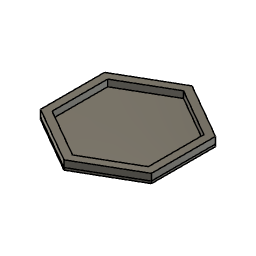
hexagon plate1 v8 (Autodesk Fusion 360 design; units mm, degrees)
Autodesk Fusion 360 part; units mm, degrees
note: some values were not read from the file. Set by a fixed rule: which sketch regions a step uses.
sketch "bottom of the plate" plane through (0, 0, 0) normal (0, 1, 0) x (1, 0, 0)
  line L0 (-150, -86.6025) -> (0, -173.2051)
  line L1 (0, -173.2051) -> (150, -86.6025)
  line L2 (150, -86.6025) -> (150, 86.6025)
  line L3 (150, 86.6025) -> (0, 173.2051)
  line L4 (0, 173.2051) -> (-150, 86.6025)
  line L5 (-150, 86.6025) -> (-150, -86.6025)
  line L6 (-150, 86.6025) -> (0, 0)
  line L7 (0, 0) -> (150, 86.6025)
  line L8 (0, 0) -> (0, -173.2051)
  dimension "d1" = 300
  dimension "d2" = 346.4102
  constraint coincident L6.end L7.start
  measures "d1" distance of L2 L5
  measures "d2" distance of L0.end L3.end
extrude "Extrude1" add sketch "bottom of the plate" along normal blind 6 makes body 1
sketch "sidePart" plane through (0, 6, 0) normal (0, 1, 0) x (-1, 0, 0)
  line L0 (150, -86.6025) -> (150, 86.6025)
  line L1 (150, 86.6025) -> (0, 173.2051)
  line L2 (0, 173.2051) -> (-150, 86.6025)
  line L3 (-150, 86.6025) -> (-150, -86.6025)
  line L4 (-150, -86.6025) -> (0, -173.2051)
  line L5 (0, -173.2051) -> (150, -86.6025)
  line L6 (-325.0555, -130) -> (-174.9445, -130)
  line L7 (-336.6025, -150) -> (-163.3975, -150)
  line L8 (-336.6025, -150) -> (-325.0555, -130)
  line L9 (-163.3975, -150) -> (-174.9445, -130)
extrude "Extrude2" add sketch "sidePart" along normal blind 6 separate body contours L0 L1 L2 L3 L4 L5 makes body 2
sketch "side" plane through (0, 6, 0) normal (0, 1, 0) x (-1, 0, 0)
  line L0 (-130, -75.0555) -> (0, -150.1111)
  line L1 (0, -150.1111) -> (130, -75.0555)
  line L2 (130, -75.0555) -> (130, 75.0555)
  line L3 (130, 75.0555) -> (0, 150.1111)
  line L4 (0, 150.1111) -> (-130, 75.0555)
  line L5 (-130, 75.0555) -> (-130, -75.0555)
  line L6 (-150, -86.6025) -> (0, -173.2051)
  line L7 (0, -173.2051) -> (150, -86.6025)
  line L8 (150, -86.6025) -> (150, 86.6025)
  line L9 (150, 86.6025) -> (0, 173.2051)
  line L10 (0, 173.2051) -> (-150, 86.6025)
  line L11 (-150, 86.6025) -> (-150, -86.6025)
  dimension "d9" = 130
  measures "d9" distance of origin L5
extrude "Extrude3" add sketch "side" along normal blind 12 bodies 1
sketch "Sketch5" plane through (-65, 0, 112.5833) normal (0.5, 0, -0.866025) x (-0.866025, 0, -0.5)
  line L0 (-75.0555, 6) -> (75.0555, 6)
  line L1 (75.0555, 6) -> (75.0555, 18)
  line L2 (75.0555, 18) -> (-75.0555, 18)
  line L3 (-75.0555, 18) -> (-75.0555, 6)
  dimension "d12" = 8
sketch "Sketch6" plane through (75, 0, -129.9038) normal (0.5, 0, -0.866025) x (-0.866025, 0, -0.5)
  line L0 (-86.6025, 0) -> (86.6025, 0)
  line L1 (86.6025, 0) -> (86.6025, 18)
  line L2 (86.6025, 18) -> (-86.6025, 18)
  line L3 (-86.6025, 18) -> (-86.6025, 0)
  dimension "d13" = 12
move_face "OffsetFaces1" offset 70 1 faces at (50, 18, -136.6396) on bodies 1
sketch "Sketch7" plane through (-130, 0, 0) normal (1, 0, 0) x (0, 0, -1)
  line L0 (-75.0555, 6) -> (75.0555, 6)
  line L1 (75.0555, 6) -> (75.0555, 88)
  line L2 (75.0555, 88) -> (-75.0555, 88)
  line L3 (-75.0555, 88) -> (-75.0555, 6)
  line L4 (-173.2051, 88) -> (-86.6025, 88)
  line L5 (-173.2051, 0) -> (-86.6025, 0)
  line L6 (-173.2051, 0) -> (-173.2051, 88)
  line L7 (173.2051, 0) -> (173.2051, 88)
  dimension "d15" = 17
  dimension "d16" = 346.4102
  measures "d16" distance of L6 L7
sketch "all_sides" plane through (0, 12, 0) normal (0, 1, 0) x (-1, 0, 0)
  line L0 (0, -173.2051) -> (150, -86.6025)
  line L1 (150, -86.6025) -> (150, 86.6025)
  line L2 (150, 86.6025) -> (0, 173.2051)
  line L3 (0, 173.2051) -> (-150, 86.6025)
  line L4 (-150, 86.6025) -> (-150, -86.6025)
  line L5 (-150, -86.6025) -> (0, -173.2051)
  line L6 (150, 86.6025) -> (0, 173.2051)
  line L7 (0, 173.2051) -> (0, 150.2051)
  line L8 (150, 86.6025) -> (130.0814, 75.1025)
  line L9 (150, 86.6025) -> (173, 86.6025) construction
  line L10 (130.0814, 75.1025) -> (0, 150.2051)
  line L11 (-150, 86.6025) -> (-130.0814, 75.1025)
  line L12 (0, 173.2051) -> (-150, 86.6025)
  line L13 (0, 173.2051) -> (-150, 86.6025)
  line L14 (0, 150.2051) -> (-130.0814, 75.1025)
  line L15 (0, 173.2051) -> (0, 150.2051)
  line L16 (0, 173.2051) -> (11.5, 193.1237) construction
  line L17 (-150, -86.6025) -> (-130.0814, -75.1025)
  line L18 (-150, 86.6025) -> (-150, -86.6025)
  line L19 (-150, 86.6025) -> (-150, -86.6025)
  line L20 (-130.0814, 75.1025) -> (-130.0814, -75.1025)
  line L21 (-150, 86.6025) -> (-130.0814, 75.1025)
  line L22 (-150, 86.6025) -> (-161.5, 106.5211) construction
  line L23 (0, -173.2051) -> (0, -150.2051)
  line L24 (-150, -86.6025) -> (0, -173.2051)
  line L25 (-150, -86.6025) -> (0, -173.2051)
  line L26 (-130.0814, -75.1025) -> (0, -150.2051)
  line L27 (-150, -86.6025) -> (-130.0814, -75.1025)
  line L28 (-150, -86.6025) -> (-173, -86.6025) construction
  line L29 (150, -86.6025) -> (130.0814, -75.1025)
  line L30 (0, -173.2051) -> (150, -86.6025)
  line L31 (0, -173.2051) -> (150, -86.6025)
  line L32 (0, -150.2051) -> (130.0814, -75.1025)
  line L33 (0, -173.2051) -> (0, -150.2051)
  line L34 (0, -173.2051) -> (-11.5, -193.1237) construction
  line L35 (150, 86.6025) -> (130.0814, 75.1025)
  line L36 (150, -86.6025) -> (150, 86.6025)
  line L37 (150, -86.6025) -> (150, 86.6025)
  line L38 (130.0814, -75.1025) -> (130.0814, 75.1025)
  line L39 (150, -86.6025) -> (130.0814, -75.1025)
  line L40 (150, -86.6025) -> (161.5, -106.5211) construction
  dimension "d18" = 23
  dimension "d19" = 150
  dimension "d20" = 23
  dimension "d22" = 360
  constraint coincident L1.end L2.start
  constraint coincident L2.end L3.start
  constraint parallel L1 L7
  constraint horizontal L9
  measures "d18" distance of L2.end L7.end
extrude "Extrude4" add sketch "all_sides" along normal blind 18 separate body contours L0 L23 L29 L30 L31 L32 L33 L39 | L5 L17 L23 L24 L25 L26 L27 L33 | L1 L8 L29 L35 L36 L37 L38 L39 | L4 L11 L17 L18 L19 L20 L21 L27 | L2 L6 L7 L8 L10 L15 L35 | L3 L7 L11 L12 L13 L14 L15 L21 makes body 3
hidden bodies 1
equation "material_thikness = 6 mm"
equation "d4 = material_thikness"
equation "d7 = material_thikness"
equation "d10 = 2 * material_thikness"
equation "wall_height = material_thikness * 3"
equation "d23 = wall_height"
named bodies: "big_walls", "bottom", "walls"
